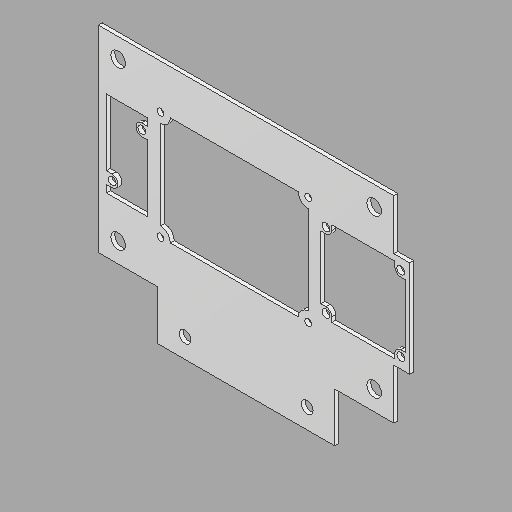
# Autodesk Inventor part: MOUNTING_PLATE
Saved by Autodesk Inventor 2025.2 (Build 292293000, 293)
## iProperties
Created: 2026-07-18
Part Number: MOUNTING_PLATE
Material: ABS Plastic
Document SubType Name: Modeling
Designer: Ben
Density: 1.06 g/cm^3
Appearance: Smooth - White
Mass: 22.6065 g
Surface Area: 240.938 cm^2
Volume: 21.3269 cm^3
Author: Ben
Autodesk Inventor part; units mm, degrees
ref_plane "YZ Plane" through (0, 0, 0) normal (1, 0, 0) x (0, 1, 0)
ref_plane "XZ Plane" through (0, 0, 0) normal (0, 1, 0) x (-1, 0, 0)
ref_plane "XY Plane" through (0, 0, 0) normal (0, 0, 1) x (1, 0, 0)
sketch "Sketch1" plane through (0, 0, 0) normal (0, 0, 1) x (1, 0, 0)
  line L0 (-75, 50) -> (75, 50)
  line L1 (75, 50) -> (75, -50)
  line L2 (75, -50) -> (-75, -50)
  line L3 (-75, -50) -> (-75, 50)
  line L4 (-75, 50) -> (75, -50) construction
  line L5 (75, 50) -> (-75, -50) construction
  line L6 (0, -100) -> (0, 75) projected
  line L7 (-106.6, 0) -> (114.6, 0) projected
  circle A0 centre (-65, 40) radius 3.75
  circle A1 centre (65, 40) radius 3.75
  circle A2 centre (65, -40) radius 3.75
  circle A3 centre (-65, -40) radius 3.75
  circle A4 centre (-31, -65) radius 3
  circle A5 centre (31, -65) radius 3
  line L8 (-45, -50) -> (-45, -75)
  line L9 (-45, -75) -> (45, -75)
  line L10 (45, -75) -> (45, -50)
  circle A6 centre (-43.5, 27.5) radius 1.75
  circle A7 centre (-43.5, -27.5) radius 1.75
  circle A8 centre (31.5, 27.5) radius 1.75
  circle A9 centre (31.5, -27.5) radius 1.75
  arc A10 (-43.5, 22.5) -> (-38.5, 27.5) centre (-43.5, 27.5) ccw
  arc A11 (-38.5, -27.5) -> (-43.5, -22.5) centre (-43.5, -27.5) ccw
  line L11 (-43.5, 22.5) -> (-43.5, -22.5)
  arc A12 (26.5, 27.5) -> (31.5, 22.5) centre (31.5, 27.5) ccw
  line L12 (-38.5, 27.5) -> (26.5, 27.5)
  arc A13 (31.5, -22.5) -> (26.5, -27.5) centre (31.5, -27.5) ccw
  line L13 (31.5, 22.5) -> (31.5, -22.5)
  line L14 (-38.5, -27.5) -> (26.5, -27.5)
  circle A14 centre (-53, 15) radius 2
  circle A15 centre (-68, -15) radius 2
  line L15 (-71, -21.75) -> (-50, -21.75)
  line L16 (-50, -21.75) -> (-50, 21.75)
  line L17 (-50, 21.75) -> (-71, 21.75)
  line L18 (-71, -21.75) -> (-50, 21.75) construction
  line L19 (-50, -21.75) -> (-71, 21.75) construction
  line L20 (-53, 15) -> (-53, -15) construction
  line L21 (-53, -15) -> (-68, -15) construction
  line L22 (-53, 15) -> (-53, -15) construction
  line L23 (-71, 21.75) -> (-71, -21.75)
  arc A16 (-68, -18) -> (-68, -12) centre (-68, -15) ccw
  arc A17 (-53, 18) -> (-53, 12) centre (-53, 15) ccw
  line L24 (-68, -12) -> (-71, -12)
  line L25 (-68, -18) -> (-71, -18)
  line L26 (-53, 12) -> (-50, 12)
  line L27 (-53, 18) -> (-50, 18)
  line L28 (38, -21.5) -> (81, -21.5)
  line L29 (81, -21.5) -> (81, 21.5)
  line L30 (81, 21.5) -> (38, 21.5)
  line L31 (38, 21.5) -> (38, -21.5)
  line L32 (38, -21.5) -> (81, 21.5) construction
  line L33 (81, -21.5) -> (38, 21.5) construction
  line L34 (75, 24.5) -> (83, 24.5)
  line L35 (83, 24.5) -> (83, -24.5)
  line L36 (83, -24.5) -> (75, -24.5)
  circle A18 centre (40.5, 19) radius 2
  circle A19 centre (78.5, 19) radius 2
  circle A20 centre (40.5, -19) radius 2
  circle A21 centre (78.5, -19) radius 2
  arc A22 (40.5, 16) -> (43.5, 19) centre (40.5, 19) ccw
  arc A23 (75.5, 19) -> (78.5, 16) centre (78.5, 19) ccw
  arc A24 (78.5, -16) -> (75.5, -19) centre (78.5, -19) ccw
  arc A25 (43.5, -19) -> (40.5, -16) centre (40.5, -19) ccw
  line L37 (43.5, 19) -> (43.5, 21.5)
  line L38 (40.5, 16) -> (38, 16)
  line L39 (75.5, 19) -> (75.5, 21.5)
  line L40 (78.5, 16) -> (81, 16)
  line L41 (78.5, -16) -> (81, -16)
  line L42 (75.5, -19) -> (75.5, -21.5)
  line L43 (43.5, -19) -> (43.5, -21.5)
  line L44 (40.5, -16) -> (38, -16)
  point P0 (0, 0)
  point P1 (0, -27.5)
  point P2 (-60.5, 0)
  point P3 (-60.5, 21.75)
  point P4 (-60.5, -15)
  point P5 (-50, 0)
  point P6 (-53, 0)
  point P7 (-43.5, 0)
  point P8 (-75, 0)
  point P9 (-71, 0)
  point P10 (59.5, 0)
  point P11 (83, 0)
  point P12 (75, 0)
  point P13 (38, 0)
  point P14 (31.5, 0)
  dimension "d0" = 100
  dimension "d1" = 150
  dimension "d4" = 7.5
  dimension "d5" = 130
  dimension "d6" = 80
  dimension "d7" = 62
  dimension "d8" = 6
  dimension "d13" = 25
  dimension "d14" = 90
  dimension "d15" = 10
  dimension "d16" = 55
  dimension "d17" = 75
  dimension "d18" = 3.5
  dimension "d19" = 5
  dimension "d20" = 5
  dimension "d22" = 43.5
  dimension "d23" = 30
  dimension "d24" = 4
  dimension "d28" = 21
  dimension "d29" = 43.5
  dimension "d30" = 4
  dimension "d31" = 15
  dimension "d32" = 3
  dimension "d33" = 3
  dimension "d34" = 43
  dimension "d35" = 8
  dimension "d36" = 49
  dimension "d37" = 2
  dimension "d38" = 2.5
  dimension "d39" = 4
  dimension "d40" = 3
  constraints: 86 end point, 28 point on line, 26 centre point, 20 point on circle, 20 vertical alignment, 18 perpendicular, 17 horizontal alignment, 17 midpoint, 12 coincident, 10 equal radius, 7 equal length, 5 horizontal, 4 vertical, 6 other
  measures "d0" distance of L2.end L0.start
  measures "d1" distance of L0.start L0.end
  measures "d4" diameter of A0
  measures "d5" distance of A1.centre A0.centre
  measures "d6" distance of A0.centre A3.centre
  measures "d7" distance of A5.centre A4.centre
  measures "d8" diameter of A4
  measures "d13" distance between parallel lines of L9 L2
  measures "d14" distance between parallel lines of L10 L8
  measures "d15" distance from line of L9 A5.centre
  measures "d16" distance of A9.centre A8.centre
  measures "d17" distance of A8.centre A6.centre
  measures "d18" diameter of A6
  measures "d19" distance of L12.start A6.centre
  measures "d20" distance of A8.centre L12.end
  measures "d22" distance from line of point (0, -27.5) L11
  measures "d23" vertical distance of A15.centre A14.centre
  measures "d24" diameter of A14
  measures "d28" distance of L16.end L17.end
  measures "d29" distance of L15.end L16.end
  measures "d30" distance between parallel lines of L3 L23
  measures "d31" horizontal distance of A15.centre A14.centre
  measures "d32" distance of L21.end L24.start
  measures "d33" distance of A14.centre L27.start
  measures "d34" distance of L29.end L30.end
  measures "d35" distance between parallel lines of L1 L35
  measures "d36" distance of L34.end L35.end
  measures "d37" distance between parallel lines of L35 L29
  measures "d38" distance from line of L29 A19.centre
  measures "d39" diameter of A19
  measures "d40" distance of L38.start A22.centre
extrude "Extrusion1" add sketch "Sketch1" along normal blind 2 contours L0 L6 L12 A10 L11 L7 L16 L17 L23 L3 | L0 L1 L30 L31 L7 L13 A12 L12 L6 | L7 L23 L15 L16 L11 A11 L14 L6 L2 L3 | L34 L35 L7 L29 L30 L1 | L2 L6 L9 L8 | L24 A16 L25 L23 | L14 A13 L13 L7 L31 L28 L1 L2 L6 | L2 L10 L9 L6 | L26 A17 L27 L16 | L30 L29 L40 A23 L39 | L37 A22 L38 L31 L30 | L35 L36 L1 L28 L29 L7 | L44 A25 L43 L28 L31 | L42 A24 L41 L29 L28
body "Solid1"
